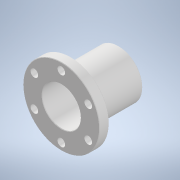
# Autodesk Inventor part: TungstenFlange
Saved by Autodesk Inventor 2020 (Build 240168000, 168)
## iProperties
Created: 2019-09-29
Part Number: TungstenFlange
Material: Generic
Document SubType Name: Modeling
Designer: vmiguel
Density: 1 g/cm^3
Appearance: Default
Author: vmiguel
Autodesk Inventor part; units mm, degrees
ref_plane "YZ Plane" through (0, 0, 0) normal (1, 0, 0) x (0, 1, 0)
ref_plane "XZ Plane" through (0, 0, 0) normal (0, 1, 0) x (-1, 0, 0)
ref_plane "XY Plane" through (0, 0, 0) normal (0, 0, 1) x (1, 0, 0)
sketch "Sketch1" plane through (0, 0, 0) normal (0, 1, 0) x (-1, 0, 0)
  line L0 (8.2, 0) -> (19.8, 0)
  line L1 (20, -0.2) -> (20, -3.8)
  line L2 (19.8, -4) -> (10, -4)
  line L3 (10, -4) -> (10, -23.8)
  line L4 (8, -23.8) -> (8, -0.2)
  line L5 (0, 0) -> (0, -60.12)
  line L6 (9.8, -24) -> (8.2, -24)
  line L7 (20, -0.2) -> (19.8, 0)
  line L8 (20, -3.8) -> (19.8, -4)
  line L9 (8.2, 0) -> (8, -0.2)
  line L10 (8, -23.8) -> (8.2, -24)
  line L11 (9.8, -24) -> (10, -23.8)
  point P0 (8, 0)
  point P1 (20, 0)
  point P2 (20, -4)
  point P3 (10, -24)
  point P4 (8, -24)
  dimension "d0" = 40
  dimension "d1" = 4
  dimension "d2" = 20
  dimension "d6" = 10
  dimension "d7" = 2
  dimension "d8" = 20
  dimension "d9" = 16
  dimension "d10" = 0.2
  dimension "d11" = 0.2
  dimension "d12" = 0.2
  dimension "d13" = 0.2
  dimension "d14" = 0.2
  dimension "d15" = 0.2
  dimension "d16" = 0.2
  dimension "d17" = 0.2
  dimension "d18" = 0.2
  dimension "d19" = 0.2
  constraints: 24 end point, 10 point on line, 4 perpendicular, 2 horizontal, 1 horizontal alignment, 1 vertical
  measures "d0" diameter of L1 L5
  measures "d1" distance of point (20, 0) point (20, -4)
  measures "d2" distance of L2.end point (10, -24)
  measures "d6" distance of point (20, -4) L2.end
  measures "d7" distance between parallel lines of L3 L4
  measures "d8" diameter of L3 L5
  measures "d9" diameter of L4 L5
  measures "d10" distance of L1.start point (20, 0)
  measures "d11" distance of L0.end point (20, 0)
  measures "d12" distance of L1.end point (20, -4)
  measures "d13" distance of L2.start point (20, -4)
  measures "d14" distance of L0.start point (8, 0)
  measures "d15" distance of L4.end point (8, 0)
  measures "d16" distance of L4.start point (8, -24)
  measures "d17" distance of L6.end point (8, -24)
  measures "d18" distance of L6.start point (10, -24)
  measures "d19" distance of L3.end point (10, -24)
revolve "Revolution1" add sketch "Sketch1" angle 360 about axis through (0, 0, 0) along (0, 0, -1)
sketch "Sketch2" plane through (0, 0, 0) normal (0, 0, 1) x (1, 0, 0)
  circle A0 centre (0, 0) radius 20 projected
  point P0 (0, 16)
  dimension "d21" = 16
  constraints: 1 vertical alignment
  measures "d21" distance of A0.centre point (0, 16)
hole "Hole1" at (0, 16, 0) direction (0, 0, -1) diameter 3.2 end through all
pattern_circular "Circular Pattern1" count 6 over 360 about axis through (0, 0, -2) along (0, 0, -1) of "Hole1"
equation "\"d11\" = d10"
equation "\"d12\" = d10"
equation "\"d13\" = d12"
equation "\"d14\" = d10"
equation "\"d15\" = d14"
equation "\"d16\" = d10"
equation "\"d17\" = d16"
equation "\"d18\" = d10"
equation "\"d19\" = d18"
body "Solid1"
